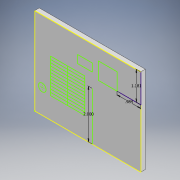
# Autodesk Inventor part: compnent box front
Saved by Autodesk Inventor 2021 (Build 250183000, 183)
## iProperties
Created: 2023-04-24
Part Number: compnent box front
Material: Generic
Document SubType Name: Modeling
Designer: boyle
Density: 1 g/cm^3
Appearance: Default
Author: boyle
Autodesk Inventor part; units mm, degrees
ref_plane "YZ Plane" through (0, 0, 0) normal (1, 0, 0) x (0, 1, 0)
ref_plane "XZ Plane" through (0, 0, 0) normal (0, 1, 0) x (-1, 0, 0)
ref_plane "XY Plane" through (0, 0, 0) normal (0, 0, 1) x (1, 0, 0)
sketch "Sketch1" plane through (0, 0, 0) normal (0, 0, 1) x (1, 0, 0)
  line L0 (0, 0) -> (111.76, 0)
  line L1 (111.76, 0) -> (111.76, 91.44)
  line L2 (111.76, 91.44) -> (0, 91.44)
  line L3 (0, 91.44) -> (0, 0)
  dimension "d0" = 111.76
  dimension "d1" = 91.44
  constraints: 8 end point, 2 parallel, 1 horizontal, 1 perpendicular
  measures "d0" distance of L2.end L1.end
  measures "d1" distance of L1.end L0.end
extrude "Extrusion1" add sketch "Sketch1" along normal blind 4.826
sketch "Sketch2" plane through (0, 0, 4.826) normal (0, 0, 1) x (1, 0, 0)
  line L0 (111.76, 0) -> (111.76, 91.44) projected
  line L1 (111.76, 91.44) -> (0, 91.44) projected
  line L2 (0, 91.44) -> (0, 0) projected
  line L3 (0, 0) -> (111.76, 0) projected
  line L4 (34.5493, 37.338) -> (52.5493, 37.338)
  line L5 (52.5493, 40.338) -> (16.5493, 40.338)
  line L6 (16.5493, 43.338) -> (52.5493, 43.338)
  line L7 (34.5493, 46.338) -> (52.5493, 46.338)
  line L8 (16.5493, 49.338) -> (52.5493, 49.338)
  line L9 (52.5493, 52.338) -> (16.5493, 52.338)
  line L10 (34.5493, 55.338) -> (52.5493, 55.338)
  line L11 (16.5493, 58.338) -> (52.5493, 58.338)
  line L12 (16.5493, 58.338) -> (16.5493, 22.338)
  line L13 (52.5493, 22.338) -> (16.5493, 22.338)
  line L14 (34.5493, 25.338) -> (52.5493, 25.338)
  line L15 (34.5493, 28.338) -> (52.5493, 28.338)
  line L16 (34.5493, 31.338) -> (52.5493, 31.338)
  line L17 (34.5493, 34.338) -> (52.5493, 34.338)
  line L18 (66.96, 79.167) -> (86.76, 79.167)
  line L19 (66.96, 61.44) -> (66.96, 79.167)
  line L20 (86.76, 61.44) -> (66.96, 61.44)
  line L21 (86.76, 79.167) -> (86.76, 61.44)
  line L22 (60.6088, 74.0565) -> (60.6088, 65.8015)
  line L23 (60.6088, 65.8015) -> (45.0584, 65.8015)
  line L24 (45.0584, 65.8015) -> (45.0584, 74.0565)
  line L25 (45.0584, 74.0565) -> (60.6088, 74.0565)
  circle A0 centre (7.874, 25.4) radius 4.0005
  line L26 (66.96, 79.167) -> (86.76, 79.167)
  line L27 (86.76, 79.167) -> (86.76, 61.44)
  line L28 (86.76, 61.44) -> (66.96, 61.44)
  line L29 (66.96, 61.44) -> (66.96, 79.167)
  line L30 (52.5493, 58.338) -> (16.5493, 58.338)
  line L31 (16.5493, 58.338) -> (16.5493, 22.338)
  line L32 (16.5493, 22.338) -> (52.5493, 22.338)
  line L33 (52.5493, 22.338) -> (52.5493, 58.338)
  circle A1 centre (7.874, 25.4) radius 4.0005
  line L34 (34.5493, 58.338) -> (34.5493, 22.338)
  line L35 (16.5493, 55.338) -> (52.5493, 55.338)
  line L36 (52.5493, 52.338) -> (16.5493, 52.338)
  line L37 (16.5493, 49.338) -> (52.5493, 49.338)
  line L38 (52.5493, 46.338) -> (16.5493, 46.338)
  line L39 (16.5493, 43.338) -> (52.5493, 43.338)
  line L40 (52.5493, 40.338) -> (16.5493, 40.338)
  line L41 (16.5493, 37.338) -> (52.5493, 37.338)
  line L42 (52.5493, 34.338) -> (16.5493, 34.338)
  line L43 (16.5493, 31.338) -> (52.5493, 31.338)
  line L44 (52.5493, 28.338) -> (16.5493, 28.338)
  line L45 (16.5493, 25.338) -> (52.5493, 25.338)
  line L46 (60.6088, 0) -> (60.6088, 50.8)
  line L47 (111.76, 91.44) -> (111.76, 61.44)
  line L48 (111.76, 61.44) -> (86.76, 61.44)
  line L49 (86.76, 79.167) -> (86.76, 61.44)
  dimension "d4" = 50.8
  dimension "d7" = 30
  dimension "d8" = 25
  constraints: 90 end point, 5 collinear, 5 horizontal, 5 parallel, 4 perpendicular, 2 centre point, 2 coincident, 2 midpoint, 2 vertical, 1 concentric, 1 point on line, 10 other
  measures "d4" distance of L46.start L46.end
  measures "d7" distance of L0.end L47.end
  measures "d8" distance of L47.end L48.end
body "Solid1"
